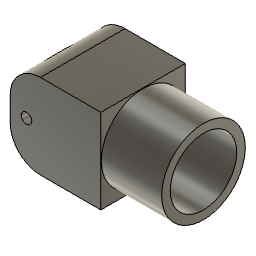
h2_case (Autodesk Fusion 360 archive; units mm, degrees)
design "mount_v2"
Autodesk Fusion 360 part; units mm, degrees
sketch "Sketch6" plane through (0, 0, 0) normal (1, 0, 0) x (0, 1, 0)
  circle A0 centre (0, 0) radius 13.825
  circle A1 centre (0, 0) radius 11
  line L0 (-14, 14) -> (14, 14)
  line L1 (14, 14) -> (14, -14)
  line L2 (14, -14) -> (-14, -14)
  line L3 (-14, -14) -> (-14, 14)
  line L4 (-14, 14) -> (14, -14) construction
  line L5 (14, 14) -> (-14, -14) construction
  dimension "d41" = 27.65
  dimension "d42" = 22
  constraint coincident A0.centre A1.centre
  constraint concentric A0 A1
  constraint horizontal L0
  constraint perpendicular L0 L1
  constraint parallel L0 L2
  constraint parallel L1 L3
  constraint coincident L4 A0.centre
  constraint coincident L5 A0.centre
  measures "d41" diameter of A0
  measures "d42" diameter of A1
extrude "Extrude8" add sketch "Sketch6" along normal blind 20 contours A0
extrude "Extrude9" add sketch "Sketch6" against normal blind 30 contours A0 | L0 L1 L2 L3
fillet "Fillet1" radius 10 1 edges at (-30, 0, 14)
fillet "Fillet2" radius 10 1 edges at (-30, 0, -14)
sketch "Sketch7" plane through (0, 14, 0) normal (0, 1, 0) x (-1, 0, 0)
  arc A0 (20, -14) -> (30, -4) centre (20, -4) ccw
  line L0 (30, -4) -> (30, 4)
  arc A1 (30, 4) -> (20, 14) centre (20, 4) ccw
  line L1 (20, 14) -> (0, 14)
  line L2 (0, 14) -> (0, -14)
  line L3 (0, -14) -> (20, -14)
  line L4 (0, 14) -> (27.0711, -11.0711) construction
  circle A2 centre (24.6168, 0) radius 1.75
  line L5 (0, -14) -> (27.0711, 11.0711) construction
  line L6 (15.1168, 0) -> (24.6168, 0) construction
  dimension "d51" = 3.5
  dimension "d55" = 9.5
  constraint coincident L1.end L2.start
  constraint midpoint A0 L4.end
  constraint coincident L2.end L3.start
  constraint midpoint A1 L5.end
  constraint coincident L4 L6.start
  constraint coincident L5 L6.start
  constraint horizontal L6
  constraint coincident A2.centre L6.end
  measures "d51" diameter of A2
  measures "d55" distance of L6.start A2.centre
extrude "Extrude10" cut sketch "Sketch7" along normal mid plane 42 from surface at -14 contours A2
